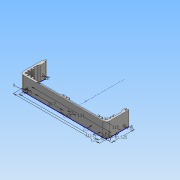
# Autodesk Inventor part: SZOMK-AK-C-C10
Saved by Autodesk Inventor 2016 (Build 200138000, 138)
## iProperties
Created: 2016-03-29
Part Number: SZOMK-AK-C-C10
Material: Generic
Document SubType Name: Modeling
Designer: admin
Density: 1 g/cm^3
Appearance: Default
d0: 120.000 mm
d1: 115.000 mm
d2: 2.100 mm
d11: 2.000 mm
d13: 39.700 mm
d14: 2.300 mm
d15: 31.200 mm
d16: 4.500 mm
d18: 115.000 mm
d19: 7.300 mm
d20: 8.400 mm
d21: 115.000 mm
d22: 111.000 mm
d23: 9.000 mm
d25: 3.000 mm
d26: 7.300 mm
d28: 1.500 mm
d29: 1.000 mm
d31: 1.500 mm
d32: 2.000 mm
d33: 2.000 mm
d34: 1.500 mm
d35: 31.525 mm
d36: 2.000 mm
d37: 1.500 mm
d38: 2.000 mm
d39: 20.000 mm
d40: 0.00 deg
d17: 10.000 mm
Author: admin
Autodesk Inventor part; units mm, degrees
ref_plane "YZ Plane" through (0, 0, 0) normal (1, 0, 0) x (0, 1, 0)
ref_plane "XZ Plane" through (0, 0, 0) normal (0, 1, 0) x (-1, 0, 0)
ref_plane "XY Plane" through (0, 0, 0) normal (0, 0, 1) x (1, 0, 0)
sketch "Sketch1" plane through (0, 0, 0) normal (0, 0, 1) x (1, 0, 0)
  line L0 (60, 0) -> (60, -27.025)
  line L1 (-60, -27.025) -> (-60, 0)
  line L2 (0, 54.7321) -> (0, -29.5526) construction
  line L3 (-1, -29.225) -> (-1, -27.025)
  line L4 (-1, -27.025) -> (1, -27.025)
  line L5 (1, -27.025) -> (1, -29.225)
  line L6 (-5, -29.225) -> (-5, -27.025)
  line L7 (-5, -27.025) -> (-3, -27.025)
  line L8 (-3, -27.025) -> (-3, -29.225)
  line L9 (3, -29.225) -> (3, -27.025)
  line L10 (3, -27.025) -> (5, -27.025)
  line L11 (5, -27.025) -> (5, -29.225)
  line L12 (-3, -29.225) -> (-1, -29.225)
  line L13 (1, -29.225) -> (3, -29.225)
  line L14 (-44.7, -29.225) -> (-44.7, -27.025)
  line L15 (-44.7, -27.025) -> (-46.7, -27.025)
  line L16 (-46.7, -27.025) -> (-46.7, -29.225)
  line L17 (-48.7, -29.225) -> (-48.7, -27.025)
  line L18 (-48.7, -27.025) -> (-50.7, -27.025)
  line L19 (-50.7, -27.025) -> (-50.7, -29.225)
  line L20 (-52.7, -29.225) -> (-50.7, -29.225)
  line L21 (-48.7, -29.225) -> (-46.7, -29.225)
  line L22 (-44.7, -29.225) -> (-5, -29.225)
  line L23 (44.7, -29.225) -> (44.7, -27.025)
  line L24 (44.7, -27.025) -> (46.7, -27.025)
  line L25 (46.7, -27.025) -> (46.7, -29.225)
  line L26 (48.7, -29.225) -> (48.7, -27.025)
  line L27 (48.7, -27.025) -> (50.7, -27.025)
  line L28 (50.7, -27.025) -> (50.7, -29.225)
  line L29 (5, -29.225) -> (44.7, -29.225)
  line L30 (46.7, -29.225) -> (48.7, -29.225)
  line L31 (50.7, -29.225) -> (52.7, -29.225)
  line L32 (-55.5, -31.525) -> (55.5, -31.525)
  line L33 (57.5, -21.825) -> (55.5, -21.825)
  line L34 (55.5, -21.825) -> (55.5, -19.825)
  line L35 (55.5, -19.825) -> (57.5, -19.825)
  line L36 (57.5, -17.825) -> (55.5, -17.825)
  line L37 (55.5, -17.825) -> (55.5, -15.825)
  line L38 (55.5, -15.825) -> (57.5, -15.825)
  line L39 (57.5, -24.225) -> (57.5, -21.825)
  line L40 (57.5, -19.825) -> (57.5, -17.825)
  line L41 (57.5, -15.825) -> (57.5, -8.1888)
  line L42 (57.5, -24.225) -> (54.9678, -24.225)
  line L43 (-57.5, -21.825) -> (-55.5, -21.825)
  line L44 (-55.5, -21.825) -> (-55.5, -19.825)
  line L45 (-55.5, -19.825) -> (-57.5, -19.825)
  line L46 (-57.5, -17.825) -> (-55.5, -17.825)
  line L47 (-55.5, -17.825) -> (-55.5, -15.825)
  line L48 (-55.5, -15.825) -> (-57.5, -15.825)
  line L49 (-57.5, -21.825) -> (-57.5, -24.225)
  line L50 (-57.5, -9.9008) -> (-57.5, -15.825)
  line L51 (-57.5, -17.825) -> (-57.5, -19.825)
  arc A0 (-60, -27.025) -> (-55.5, -31.525) centre (-55.5, -27.025) ccw
  arc A1 (55.5, -31.525) -> (60, -27.025) centre (55.5, -27.025) ccw
  arc A2 (54.0511, -26.6368) -> (55.1118, -25.5761) centre (55.5, -27.025) ccw
  arc A3 (-55.1118, -25.5761) -> (-54.0511, -26.6368) centre (-55.5, -27.025) ccw
  line L52 (52.7, -26.4928) -> (52.7, -29.225)
  line L53 (54.6142, -25.0786) -> (55.1118, -25.5761)
  line L54 (53.5536, -26.1392) -> (54.0511, -26.6368)
  line L55 (55.5, -27.025) -> (52.7, -24.225) construction
  arc A4 (54.9678, -24.225) -> (54.6142, -25.0786) centre (54.9678, -24.725) ccw
  arc A5 (53.5536, -26.1392) -> (52.7, -26.4928) centre (53.2, -26.4928) ccw
  line L56 (-57.5, -24.225) -> (-54.9678, -24.225)
  line L57 (-52.7, -26.4928) -> (-52.7, -29.225)
  line L58 (-55.5, -27.025) -> (-52.7, -24.225) construction
  line L59 (-55.1118, -25.5761) -> (-54.6142, -25.0786)
  line L60 (-54.0511, -26.6368) -> (-53.5536, -26.1392)
  arc A6 (-54.6142, -25.0786) -> (-54.9678, -24.225) centre (-54.9678, -24.725) ccw
  arc A7 (-52.7, -26.4928) -> (-53.5536, -26.1392) centre (-53.2, -26.4928) ccw
  line L61 (-57.5, -9.9008) -> (-55.5, -7.1508)
  line L62 (-55.5, -7.1508) -> (-55.5, 0)
  line L63 (57.5, -8.1888) -> (55.5, -4.7544)
  line L64 (55.5, -4.7544) -> (55.5, 0)
  arc A8 (-57, 1.3386) -> (-58.5, 1.3386) centre (-57.75, 2) ccw
  line L65 (-58.5, 0) -> (-58.5, 1.3386)
  line L66 (-57, 0) -> (-57, 1.3386)
  line L67 (-57.75, 1.7435) -> (-57.75, 0.7418) construction
  line L68 (-60, 0) -> (-58.5, 0)
  line L69 (-57, 0) -> (-55.5, 0)
  arc A9 (57, -1.3386) -> (58.5, -1.3386) centre (57.75, -2) ccw
  line L70 (57, -1.3386) -> (57, 0)
  line L71 (58.5, -1.3386) -> (58.5, 0)
  line L72 (57.75, 2.8392) -> (57.75, 0.4457) construction
  line L73 (55.5, 0) -> (57, 0)
  line L74 (58.5, 0) -> (60, 0)
  point P0 (0, 0)
  dimension "d0" = 120
  dimension "d11" = 2
  dimension "d13" = 39.7
  dimension "d14" = 2.3
  dimension "d16" = 4.5
  dimension "d17" = 10
  dimension "d19" = 7.3
  dimension "d20" = 8.4
  dimension "d21" = 115
  dimension "d22" = 111
  dimension "d23" = 9
  dimension "d25" = 3
  dimension "d26" = 7.3
  dimension "d28" = 1.5
  dimension "d29" = 1
  dimension "d31" = 1.5
  dimension "d32" = 2
  dimension "d34" = 1.5
  dimension "d35" = 31.525
  dimension "d36" = 2
  dimension "d37" = 1.5
  dimension "d38" = 2
  dimension "d41" = 111
  constraints: 151 end point, 100 perpendicular, 25 collinear, 20 point on circle, 19 point on line, 17 equal length, 12 tangent, 12 vertical, 10 centre point, 10 parallel, 6 equal radius, 6 horizontal, 3 coincident, 13 other
  measures "d0" distance between parallel lines of L0 L1
  measures "d11" distance of L9.end L10.end
  measures "d13" distance between parallel lines of L6 L14
  measures "d14" distance between parallel lines of L32 L29
  measures "d16" distance between parallel lines of L32 L27
  measures "d17" distance between parallel lines of L11 L6
  measures "d19" distance between parallel lines of L32 L42
  measures "d20" distance between parallel lines of L42 L38
  measures "d21" distance between parallel lines of L41 L50
  measures "d22" distance between parallel lines of L34 L44
  measures "d23" diameter of A0
  measures "d25" diameter of A3
  measures "d26" distance between parallel lines of L0 L52
  measures "d28" distance between parallel lines of L53 L54
  measures "d29" diameter of A4
  measures "d31" distance between parallel lines of L60 L59
  measures "d32" diameter of A8
  measures "d34" distance between parallel lines of L66 L65
  measures "d35" distance between parallel lines of L32 L74
  measures "d36" distance from line of L74 A9.centre
  measures "d37" distance between parallel lines of L71 L70
  measures "d38" distance from line of L69 A8.centre
  measures "d41" distance of A1.centre A0.centre
extrude "Extrusion1" add sketch "Sketch1" along normal blind 20
equation "\"d26\" = d19"
equation "\"d31\" = d28"
equation "\"d36\" = d32"
equation "\"d37\" = d34"
body "Solid1"
